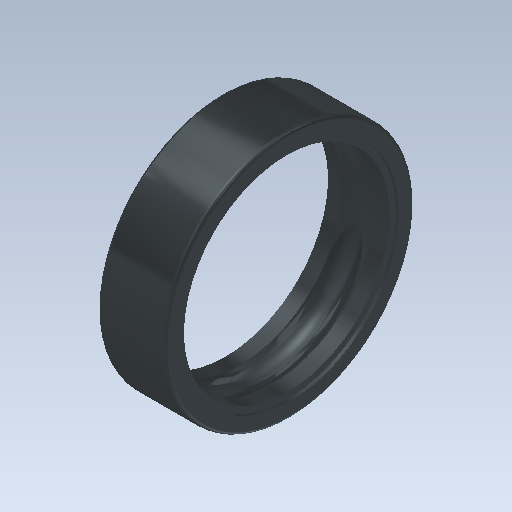
# Autodesk Inventor part: 6900ZZ Outer Ring
Saved by Autodesk Inventor 2021 (Build 250183000, 183)
## iProperties
Category: PARTsolutions
Company: NTN
Created: 2019-07-31
Part Number: 6900ZZ Outer Ring
Material: 鉄、鋳鉄
Catalog Web Link: www.cadenas.de
Description: Open type or-Deep Groove Ball Bearings
Vendor: NTN
Document SubType Name: Modeling
Designer: psadmin
Manufacturer: NTN
Mass: 4.44316 g
Surface Area: 10.1927 cm^2
Volume: 0.621421 cm^3
Density: 7.15 g/cm^3
Appearance: 鉄 灰色
PSOL_IDENT_0: {$CADENAS_DATA\23d-libs\ntn\ball_roller_bearings\deep_groove_bb\deep_groove_bb\6_types\dgbb_or.prj},
PSOL_IDENT_1: 182 {VTYP=3D},{NB=6900ZZ Outer Ring},{LINA=6900ZZ Outer Ring},{NN=Open type or},{DATE=29.01.2019 23:
PSOL_IDENT_2: 03:44},{GEOMDATE=14.01.2008 11:01:00},{VERSION=},{LINEID=2800},{WBVAR=},{WBNUMERIC=}  {NB=6900ZZ Out
PSOL_IDENT_3: er Ring},{LINA=6900ZZ Outer Ring},{KT=DUMMY},{IDNR=},{SD=10},{D=22},{B=6},{R=0.3},{ORDER1=6900},{ORD
PSOL_IDENT_4: ER=6900ZZ},{CR=2.70},{COR=1.27},{CRF=275},{CORF=129},{LSG=30000},{LSO=36000},{MASS=0.01},{RNS=0.3},{
PSOL_IDENT_5: LLH=0},{LLU=21000},{ST=ZZ},{NCST=LLB},{LTST=0},{CST=LLU},{SRG=N},{SR=NR},{D1=20.80},{A=1.05},{BA=0.8
PSOL_IDENT_6: 0},{R0=0.20},{D2=24.8},{F=0.70},{DA1=12},{DA2=13},{DA=20},{DX=25.5},{CY=1.5},{CZ=0.7},{RAS=0.3},{RNA
PSOL_IDENT_7: S=0.3},{VERS=2},{X=6},{N=8},{RB=1.80000},{O=50.24000}
NN: Open type or
NT: Deep Groove Ball Bearings
NB: 6900ZZ Outer Ring
NBSYN: $ORDER. Outer Ring
LINA: 6900ZZ Outer Ring
SD: 10
D: 22
B: 6
R: 0.3
ORDER1: 6900
CR: 2.70
COR: 1.27
CRF: 275
CORF: 129
LSG: 30000
LSO: 36000
MASS: 0.01
RNS: 0.3
LLH: 0
LLU: 21000
ST: ZZ
NCST: LLB
LTST: 0
CST: LLU
SRG: N
SR: NR
D1: 20.8
A: 1.05
BA: 0.8
R0: 0.2
D2: 0
F: 0.7
DA1: 12
DA2: 13
DA: 20
DX: 25.5
CY: 1.5
CZ: 0.7
RAS: 0.3
RNAS: 0.3
VERS: 2
SUPPLIER: NTN
ARTICLENO: 6900ZZ Outer Ring
BOMINFO: 6900ZZ Outer Ring
CREATOR: CADENAS GmbH
d3: 0.000 mm
Title: 6900ZZ Outer Ring
Author: Cadenas PARTsolutions
Comments: Deep Groove Ball Bearings
Autodesk Inventor part; units mm, degrees
sketch "Sketch_1" plane through (0, 0, 0) normal (0, 0, 1) x (1, 0, 0)
  line L0 (6, 0) -> (0, 0)
  line L1 (0, 9.08) -> (1.56, 9.08)
  arc A0 (4.44, 9.08) -> (1.56, 9.08) centre (3, 8) ccw
  line L2 (4.44, 9.08) -> (6, 9.08)
  line L3 (6, 9.08) -> (6, 10.7)
  arc A1 (6, 10.7) -> (5.7, 11) centre (5.7, 10.7) ccw
  line L4 (5.7, 11) -> (0.3, 11)
  arc A2 (0.3, 11) -> (0, 10.7) centre (0.3, 10.7) ccw
  line L5 (0, 10.7) -> (0, 9.08)
  constraints: 12 end point, 6 point on circle, 3 centre point
revolve "Revolution1" add sketch "Sketch_1" angle 360 about axis through (6, 0, 0) along (1, 0, 0)
sketch "Sketch_4" plane through (0, 0, 0) normal (0, 0, 1) x (1, 0, 0)
  line L0 (6, 0) -> (0, 0)
  line L1 (0, 9.6133) -> (0, 8)
  line L2 (0, 8) -> (6, 8)
  line L3 (6, 8) -> (6, 9.6133)
  line L4 (6, 9.6133) -> (5.724, 9.6133)
  line L5 (5.724, 9.6133) -> (5.724, 8.9)
  line L6 (5.724, 8.9) -> (0.276, 8.9)
  line L7 (0.276, 8.9) -> (0.276, 9.6133)
  line L8 (0.276, 9.6133) -> (0, 9.6133)
  constraints: 18 end point
revolve "Revolution2" cut sketch "Sketch_4" angle 360 about axis through (6, 0, 0) along (1, 0, 0)
ref_plane "dgbb_or_XY" through (0, 0, 0) normal (1, 0, 0) x (0, 0, -1)
ref_plane "dgbb_or_YZ" through (0, 0, 0) normal (0, 0, -1) x (0, 1, 0)
ref_plane "dgbb_or_ZX" through (0, 0, 0) normal (0, 1, 0) x (1, 0, 0)
ref_plane "dgbb_or1_XY" through (6, 0, 0) normal (1, 0, 0) x (0, 0, -1)
ref_plane "dgbb_or1_YZ" through (6, 0, 0) normal (0, 0, -1) x (0, 1, 0)
ref_plane "dgbb_or1_ZX" through (6, 0, 0) normal (0, 1, 0) x (1, 0, 0)
ref_plane "dgbb_or11_1_XY" through (3, 8, 0) normal (1, 0, 0) x (0, 0, -1)
ref_plane "dgbb_or11_1_YZ" through (3, 8, 0) normal (0, 0, -1) x (0, 1, 0)
ref_plane "dgbb_or11_1_ZX" through (3, 8, 0) normal (0, 1, 0) x (1, 0, 0)
ref_plane "dgbb_or11_2_XY" through (3, 5.6569, 5.6569) normal (1, 0, 0) x (0, 0, -1)
ref_plane "dgbb_or11_2_YZ" through (3, 5.6569, 5.6569) normal (0, 0, -1) x (0, 1, 0)
ref_plane "dgbb_or11_2_ZX" through (3, 5.6569, 5.6569) normal (0, 1, 0) x (1, 0, 0)
ref_plane "dgbb_or11_3_XY" through (3, 0, 8) normal (1, 0, 0) x (0, 0, -1)
ref_plane "dgbb_or11_3_YZ" through (3, 0, 8) normal (0, 0, -1) x (0, 1, 0)
ref_plane "dgbb_or11_3_ZX" through (3, 0, 8) normal (0, 1, 0) x (1, 0, 0)
ref_plane "dgbb_or11_4_XY" through (3, -5.6569, 5.6569) normal (1, 0, 0) x (0, 0, -1)
ref_plane "dgbb_or11_4_YZ" through (3, -5.6569, 5.6569) normal (0, 0, -1) x (0, 1, 0)
ref_plane "dgbb_or11_4_ZX" through (3, -5.6569, 5.6569) normal (0, 1, 0) x (1, 0, 0)
ref_plane "dgbb_or11_5_XY" through (3, -8, 0) normal (1, 0, 0) x (0, 0, -1)
ref_plane "dgbb_or11_5_YZ" through (3, -8, 0) normal (0, 0, -1) x (0, 1, 0)
ref_plane "dgbb_or11_5_ZX" through (3, -8, 0) normal (0, 1, 0) x (1, 0, 0)
ref_plane "dgbb_or11_6_XY" through (3, -5.6569, -5.6569) normal (1, 0, 0) x (0, 0, -1)
ref_plane "dgbb_or11_6_YZ" through (3, -5.6569, -5.6569) normal (0, 0, -1) x (0, 1, 0)
ref_plane "dgbb_or11_6_ZX" through (3, -5.6569, -5.6569) normal (0, 1, 0) x (1, 0, 0)
ref_plane "dgbb_or11_7_XY" through (3, 0, -8) normal (1, 0, 0) x (0, 0, -1)
ref_plane "dgbb_or11_7_YZ" through (3, 0, -8) normal (0, 0, -1) x (0, 1, 0)
ref_plane "dgbb_or11_7_ZX" through (3, 0, -8) normal (0, 1, 0) x (1, 0, 0)
ref_plane "dgbb_or11_8_XY" through (3, 5.6569, -5.6569) normal (1, 0, 0) x (0, 0, -1)
ref_plane "dgbb_or11_8_YZ" through (3, 5.6569, -5.6569) normal (0, 0, -1) x (0, 1, 0)
ref_plane "dgbb_or11_8_ZX" through (3, 5.6569, -5.6569) normal (0, 1, 0) x (1, 0, 0)
body "Solid1"
